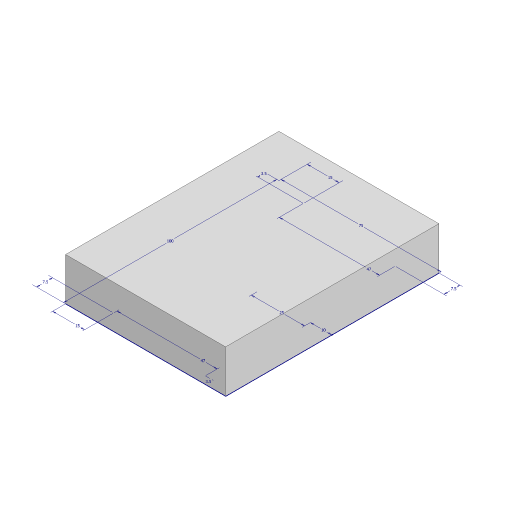
# Autodesk Inventor part: 2x-servo-boards-QS-series
Saved by Autodesk Inventor 2023 (Build 270158000, 158)
## iProperties
Created: 2024-08-27
Part Number: 2x-servo-boards-QS-series
Material: Generic
Document SubType Name: Modeling
Designer: N.Vladimirov
Density: 1 g/cm^3
Appearance: Default
Author: N.Vladimirov
Autodesk Inventor part; units mm, degrees
ref_plane "YZ Plane" through (0, 0, 0) normal (1, 0, 0) x (0, 1, 0)
ref_plane "XZ Plane" through (0, 0, 0) normal (0, 1, 0) x (-1, 0, 0)
ref_plane "XY Plane" through (0, 0, 0) normal (0, 0, 1) x (1, 0, 0)
sketch "Sketch1" plane through (0, 0, 0) normal (0, 1, 0) x (-1, 0, 0)
  line L0 (0, 0) -> (75, 0)
  line L1 (75, 0) -> (75, -100)
  line L2 (75, -100) -> (0, -100)
  line L3 (0, -100) -> (0, 0)
  point P0 (60, -7.5)
  point P1 (13, -3.5)
  point P2 (60, -96.5)
  point P3 (13, -92.5)
  point P4 (35, -50)
  point P5 (10, -50)
  point P6 (0, -50)
  dimension "d0" = 75
  dimension "d1" = 100
  dimension "d2" = 7.5
  dimension "d3" = 3.5
  dimension "d4" = 3.5
  dimension "d5" = 7.5
  dimension "d6" = 47
  dimension "d7" = 47
  dimension "d8" = 15
  dimension "d9" = 15
  dimension "d10" = 25
  dimension "d11" = 10
  constraints: 8 end point, 2 parallel, 1 horizontal, 1 midpoint, 1 perpendicular
  measures "d0" distance of L1.end L2.end
  measures "d1" distance of L0.end L1.end
  measures "d2" distance from line of L0 point (60, -7.5)
  measures "d3" distance from line of L0 point (13, -3.5)
  measures "d4" distance from line of L2 point (60, -96.5)
  measures "d5" distance from line of L2 point (13, -92.5)
  measures "d6" horizontal distance of point (13, -3.5) point (60, -7.5)
  measures "d7" horizontal distance of point (13, -92.5) point (60, -96.5)
  measures "d8" distance from line of point (60, -7.5) L1
  measures "d9" distance from line of L1 point (60, -96.5)
  measures "d10" distance of point (10, -50) point (35, -50)
  measures "d11" distance of point (0, -50) point (10, -50)
extrude "Extrusion1" add sketch "Sketch1" along normal blind 20
hole "Hole1" at (-13, 0, -3.5) at (-60, 0, -7.5) at (-13, 0, -92.5) at (-60, 0, -96.5) direction (0, 1, 0) diameter 2.459 depth 8 tip angle 118 thread size "M3x0.5" class "6H" standard "ISO Metric profile"
hole "Hole2" at (-35, 0, -50) at (-10, 0, -50) direction (0, 1, 0) diameter 4.917 depth 16 tip angle 118 thread size "M6x1" class "6H" standard "ISO Metric profile"
body "Solid1"
